Autodesk Inventor part; units mm, degrees
(part 6 of 6)
sketch "S15_195p3" plane through (0, 0, 0) normal (0, 0, 1) x (1, 0, 0)
  spline S0 degree 4 poles (125.9816, -53.0872) (125.9571, -53.0702) (125.8376, -52.9864) (125.6366, -52.8466) (125.2975, -52.6104) (124.9408, -52.3617) (124.502, -52.0575) (123.9855, -51.6987) (123.3893, -51.2867) (122.7156, -50.8212) (121.9638, -50.3042) (121.135, -49.7351) (120.2298, -49.1159) (119.2485, -48.447) (118.1926, -47.7295) (117.0618, -46.9649) (115.8579, -46.154) (114.5815, -45.2984) (113.2337, -44.3985) (111.8153, -43.4568) (110.3277, -42.474) (108.772, -41.4519) (107.1492, -40.3915) (105.4613, -39.2947) (103.7089, -38.1629) (101.8941, -36.9982) (100.0179, -35.8012) (98.0825, -34.5747) (96.0888, -33.3192) (94.0391, -32.0378) (91.9348, -30.7309) (89.7779, -29.4013) (87.5702, -28.05) (85.3138, -26.6795) (83.0104, -25.2909) (80.6627, -23.8865) (78.2717, -22.4682) (75.8404, -21.0375) (73.3708, -19.5968) (70.865, -18.1474) (68.3252, -16.6917) (65.7538, -15.2313) (63.1532, -13.7681) (60.5259, -12.3041) (57.8736, -10.8415) (55.1998, -9.382) (52.5061, -7.927) (49.7953, -6.4797) (47.0699, -5.0405) (44.3326, -3.6125) (41.5854, -2.1967) (38.8317, -0.7957) (36.073, 0.5886) (33.3129, 1.9555) (30.5532, 3.3018) (27.7948, 4.6278) (25.0442, 5.9287) (22.2894, 7.2111) (19.5352, 8.4618) (16.7929, 9.679) (14.0628, 10.861) (11.3496, 12.0056) (8.6564, 13.1126) (5.9856, 14.1789) (3.3403, 15.2059) (0.7234, 16.1899) (-1.8626, 17.1321) (-4.4145, 18.0303) (-6.9297, 18.8849) (-9.4054, 19.6941) (-11.839, 20.4583) (-14.2276, 21.1764) (-16.5684, 21.8487) (-18.8593, 22.4742) (-21.097, 23.0535) (-23.2793, 23.5858) (-25.4039, 24.072) (-27.468, 24.5112) (-29.4695, 24.9047) (-31.4059, 25.2518) (-33.2754, 25.5529) (-35.0752, 25.8094) (-36.8039, 26.0205) (-38.4591, 26.1872) (-40.0392, 26.3106) (-41.5422, 26.3902) (-42.9667, 26.4274) (-44.3109, 26.4227) (-45.5737, 26.3765) (-46.7533, 26.2893) (-47.8492, 26.1622) (-48.8598, 25.9957) (-49.7845, 25.7897) (-50.623, 25.546) (-51.3739, 25.263) (-52.0377, 24.9422) (-52.6135, 24.5832) (-53.1006, 24.185) (-53.497, 23.7471) (-53.8017, 23.2714) (-54.0117, 22.7577) (-54.1273, 22.2149) (-54.1441, 21.6505) (-54.0641, 21.0658) (-53.8887, 20.4629) (-53.6195, 19.8419) (-53.2579, 19.2032) (-52.805, 18.5459) (-52.2615, 17.8703) (-51.628, 17.1764) (-50.9052, 16.4646) (-50.094, 15.7355) (-49.1952, 14.9891) (-48.2099, 14.2264) (-47.1391, 13.4475) (-45.984, 12.6535) (-44.7459, 11.8441) (-43.4261, 11.0212) (-42.0259, 10.1841) (-40.5473, 9.334) (-38.9911, 8.4715) (-37.3595, 7.5976) (-35.6542, 6.7113) (-33.8766, 5.8153) (-32.0292, 4.9082) (-30.113, 3.9916) (-28.131, 3.0654) (-26.0847, 2.1299) (-23.9762, 1.1866) (-21.808, 0.2339) (-19.5818, -0.7255) (-17.3006, -1.6936) (-14.9662, -2.6682) (-12.581, -3.6503) (-10.1481, -4.6394) (-7.6689, -5.6346) (-5.1471, -6.6365) (-2.5846, -7.6445) (0.0159, -8.6582) (2.6516, -9.6779) (5.3196, -10.7034) (8.0177, -11.7337) (10.7442, -12.7705) (13.4952, -13.8109) (16.2737, -14.861) (19.0868, -15.914) (21.9144, -16.9645) (24.7602, -18.013) (27.6171, -19.0583) (30.4832, -20.1002) (33.3552, -21.1382) (36.2298, -22.1711) (39.1042, -23.1993) (41.9758, -24.221) (44.841, -25.2372) (47.6974, -26.2455) (50.5415, -27.247) (53.3708, -28.2398) (56.1826, -29.2234) (58.9732, -30.1979) (61.7404, -31.1616) (64.4815, -32.1139) (67.1932, -33.055) (69.873, -33.9827) (72.5183, -34.8976) (75.1261, -35.798) (77.6941, -36.6833) (80.2194, -37.5527) (82.6998, -38.4058) (85.1322, -39.2415) (87.5148, -40.0589) (89.845, -40.8572) (92.1199, -41.6363) (94.3379, -42.3942) (96.4964, -43.1316) (98.5933, -43.8466) (100.6262, -44.5396) (102.5936, -45.2086) (104.4929, -45.8543) (106.3223, -46.4752) (108.0801, -47.0711) (109.7642, -47.641) (111.373, -48.1854) (112.905, -48.7023) (114.3582, -49.1926) (115.7313, -49.6552) (117.023, -50.0894) (118.2315, -50.4956) (119.356, -50.8732) (120.395, -51.2212) (121.3472, -51.5403) (122.2122, -51.8294) (122.9882, -52.0891) (123.6752, -52.3183) (124.2717, -52.5174) (124.7779, -52.6863) (125.1907, -52.8235) (125.5826, -52.9546) (125.815, -53.0316) (125.9533, -53.0777) (125.9816, -53.0872) knots 0 0 0 0 0 0.003306 0.005253 0.00752 0.010062 0.01285 0.015861 0.019079 0.022488 0.026078 0.029837 0.033757 0.037828 0.042045 0.046398 0.050884 0.055494 0.060224 0.065069 0.070023 0.075082 0.080241 0.085495 0.090841 0.096274 0.101791 0.107386 0.113057 0.118799 0.124609 0.130484 0.136419 0.142412 0.148458 0.154554 0.160697 0.166884 0.17311 0.179374 0.185671 0.191998 0.198352 0.20473 0.211128 0.217543 0.223972 0.230412 0.23686 0.243312 0.249765 0.256217 0.262663 0.2691 0.275526 0.281941 0.288345 0.294734 0.301105 0.307451 0.313767 0.320049 0.326294 0.332498 0.338659 0.344773 0.350837 0.356848 0.362801 0.368695 0.374525 0.380288 0.38598 0.391599 0.39714 0.4026 0.407976 0.413263 0.418458 0.423557 0.428556 0.433452 0.438241 0.442917 0.447478 0.451919 0.456236 0.460425 0.464482 0.468403 0.472185 0.475825 0.479322 0.482675 0.485889 0.48897 0.49193 0.494788 0.497572 0.50031 0.503032 0.505769 0.508552 0.511409 0.514365 0.517441 0.520647 0.523991 0.527474 0.531098 0.534861 0.538758 0.542789 0.546947 0.551231 0.555634 0.560154 0.564786 0.569527 0.574371 0.579315 0.584356 0.58949 0.594712 0.60002 0.605409 0.610877 0.61642 0.622034 0.627716 0.633463 0.639271 0.645138 0.651061 0.657035 0.663059 0.669128 0.675241 0.681393 0.687582 0.693804 0.700057 0.706341 0.712655 0.718998 0.725365 0.731751 0.738149 0.744556 0.750969 0.757385 0.7638 0.770211 0.776616 0.783011 0.789393 0.795759 0.802106 0.808429 0.814727 0.820996 0.827232 0.833433 0.839595 0.845714 0.851788 0.857813 0.863785 0.869702 0.875558 0.881352 0.887078 0.892735 0.898316 0.90382 0.909242 0.914577 0.919822 0.924972 0.930023 0.93497 0.939808 0.944533 0.949139 0.95362 0.95797 0.962183 0.966252 0.970169 0.973927 0.977515 0.980924 0.984141 0.987151 0.989939 0.99248 0.994747 0.996694 1 1 1 1 1
  circle A0 centre (0, 0) radius 5.15
  line L0 (-27.08, 9.9) -> (-16.88, 9.9)
  line L1 (-16.88, 9.9) -> (-16.88, 14.1)
  line L2 (-16.88, 14.1) -> (-27.08, 14.1)
  line L3 (-27.08, 14.1) -> (-27.08, 9.9)
  line L4 (-27.08, 9.9) -> (-16.88, 14.1) construction
  line L5 (-16.88, 9.9) -> (-27.08, 14.1) construction
  line L6 (40.1, -9) -> (29.9, -9)
  line L7 (29.9, -9) -> (29.9, -13.2)
  line L8 (29.9, -13.2) -> (40.1, -13.2)
  line L9 (40.1, -13.2) -> (40.1, -9)
  line L10 (40.1, -9) -> (29.9, -13.2) construction
  line L11 (29.9, -9) -> (40.1, -13.2) construction
  point P0 (125.8216, -52.9755)
  point P1 (125.6216, -52.8361)
  point P2 (125.3419, -52.6413)
  point P3 (124.9828, -52.3912)
  point P4 (124.5442, -52.0867)
  point P5 (124.0266, -51.7276)
  point P6 (123.4303, -51.3151)
  point P7 (122.7559, -50.8495)
  point P8 (122.0038, -50.3318)
  point P9 (121.1745, -49.7626)
  point P10 (120.2687, -49.1429)
  point P11 (119.287, -48.4737)
  point P12 (118.2303, -47.7559)
  point P13 (117.0991, -46.9907)
  point P14 (115.8945, -46.1794)
  point P15 (114.6175, -45.3232)
  point P16 (113.269, -44.4231)
  point P17 (111.8498, -43.4807)
  point P18 (110.3614, -42.4974)
  point P19 (108.8049, -41.4747)
  point P20 (107.1814, -40.4137)
  point P21 (105.4925, -39.3163)
  point P22 (103.7393, -38.184)
  point P23 (101.9236, -37.0185)
  point P24 (100.0465, -35.8211)
  point P25 (98.1099, -34.5937)
  point P26 (96.1153, -33.3377)
  point P27 (94.0645, -32.0555)
  point P28 (91.9591, -30.748)
  point P29 (89.8011, -29.4175)
  point P30 (87.5924, -28.0657)
  point P31 (85.3348, -26.6943)
  point P32 (83.0303, -25.3051)
  point P33 (80.6812, -23.9)
  point P34 (78.2891, -22.4809)
  point P35 (75.8565, -21.0495)
  point P36 (73.3857, -19.608)
  point P37 (70.8786, -18.158)
  point P38 (68.3375, -16.7015)
  point P39 (65.7647, -15.2403)
  point P40 (63.1628, -13.7764)
  point P41 (60.534, -12.3118)
  point P42 (57.8805, -10.8484)
  point P43 (55.2052, -9.3881)
  point P44 (52.5101, -7.9326)
  point P45 (49.7979, -6.4844)
  point P46 (47.0711, -5.0447)
  point P47 (44.3323, -3.616)
  point P48 (41.5838, -2.1997)
  point P49 (38.8284, -0.798)
  point P50 (36.0685, 0.5871)
  point P51 (33.3069, 1.9542)
  point P52 (30.5459, 3.3012)
  point P53 (27.7884, 4.6264)
  point P54 (25.0368, 5.9279)
  point P55 (22.2802, 7.2088)
  point P56 (19.5233, 8.4612)
  point P57 (16.7777, 9.6794)
  point P58 (14.0462, 10.8618)
  point P59 (11.3315, 12.007)
  point P60 (8.6368, 13.1139)
  point P61 (5.9647, 14.181)
  point P62 (3.318, 15.2077)
  point P63 (0.6997, 16.1923)
  point P64 (-1.8875, 17.1344)
  point P65 (-4.4407, 18.0329)
  point P66 (-6.9572, 18.8874)
  point P67 (-9.4342, 19.6968)
  point P68 (-11.8691, 20.4608)
  point P69 (-14.2588, 21.179)
  point P70 (-16.6008, 21.8509)
  point P71 (-18.8928, 22.4764)
  point P72 (-21.1316, 23.0553)
  point P73 (-23.3149, 23.5875)
  point P74 (-25.4404, 24.073)
  point P75 (-27.5056, 24.512)
  point P76 (-29.5079, 24.9048)
  point P77 (-31.4452, 25.2513)
  point P78 (-33.3153, 25.5519)
  point P79 (-35.1159, 25.8073)
  point P80 (-36.8451, 26.0175)
  point P81 (-38.5008, 26.1833)
  point P82 (-40.0812, 26.3052)
  point P83 (-41.5845, 26.3837)
  point P84 (-43.0089, 26.4193)
  point P85 (-44.3529, 26.4128)
  point P86 (-45.6152, 26.3646)
  point P87 (-46.794, 26.2754)
  point P88 (-47.8885, 26.146)
  point P89 (-48.8972, 25.9768)
  point P90 (-49.8192, 25.7683)
  point P91 (-50.6537, 25.5214)
  point P92 (-51.3998, 25.2362)
  point P93 (-52.0569, 24.9136)
  point P94 (-52.6244, 24.554)
  point P95 (-53.1019, 24.1576)
  point P96 (-53.489, 23.7248)
  point P97 (-53.7859, 23.2561)
  point P98 (-53.9921, 22.7517)
  point P99 (-54.1059, 22.2187)
  point P100 (-54.125, 21.6643)
  point P101 (-54.05, 21.0889)
  point P102 (-53.8812, 20.4926)
  point P103 (-53.619, 19.8758)
  point P104 (-53.2638, 19.2391)
  point P105 (-52.8162, 18.5825)
  point P106 (-52.2772, 17.9068)
  point P107 (-51.6474, 17.2122)
  point P108 (-50.9275, 16.4994)
  point P109 (-50.1186, 15.769)
  point P110 (-49.2216, 15.0214)
  point P111 (-48.2377, 14.2573)
  point P112 (-47.1679, 13.4772)
  point P113 (-46.0136, 12.6818)
  point P114 (-44.776, 11.8714)
  point P115 (-43.4565, 11.0471)
  point P116 (-42.0566, 10.209)
  point P117 (-40.5778, 9.3578)
  point P118 (-39.0216, 8.4943)
  point P119 (-37.3897, 7.6191)
  point P120 (-35.684, 6.7323)
  point P121 (-33.9061, 5.835)
  point P122 (-32.0581, 4.9272)
  point P123 (-30.1415, 4.0095)
  point P124 (-28.1587, 3.0825)
  point P125 (-26.1117, 2.1464)
  point P126 (-24.0026, 1.2018)
  point P127 (-21.8334, 0.2488)
  point P128 (-19.6065, -0.7119)
  point P129 (-17.3243, -1.6803)
  point P130 (-14.989, -2.6559)
  point P131 (-12.6029, -3.6387)
  point P132 (-10.1688, -4.6284)
  point P133 (-7.6887, -5.6245)
  point P134 (-5.1658, -6.627)
  point P135 (-2.6021, -7.6357)
  point P136 (-0.0005, -8.6502)
  point P137 (2.6364, -9.6706)
  point P138 (5.3056, -10.6967)
  point P139 (8.0047, -11.7278)
  point P140 (10.7308, -12.7643)
  point P141 (13.4812, -13.8054)
  point P142 (16.2622, -14.8546)
  point P143 (19.0767, -15.9086)
  point P144 (21.9086, -16.9605)
  point P145 (24.7556, -18.0098)
  point P146 (27.6142, -19.0558)
  point P147 (30.4816, -20.0984)
  point P148 (33.355, -21.1369)
  point P149 (36.2311, -22.1706)
  point P150 (39.107, -23.1991)
  point P151 (41.9798, -24.2218)
  point P152 (44.8466, -25.2382)
  point P153 (47.7044, -26.2475)
  point P154 (50.55, -27.2493)
  point P155 (53.3807, -28.2427)
  point P156 (56.1939, -29.227)
  point P157 (58.986, -30.2018)
  point P158 (61.7546, -31.1661)
  point P159 (64.497, -32.1191)
  point P160 (67.2103, -33.0604)
  point P161 (69.8914, -33.9889)
  point P162 (72.538, -34.9041)
  point P163 (75.1473, -35.805)
  point P164 (77.7165, -36.6908)
  point P165 (80.2432, -37.5607)
  point P166 (82.7249, -38.4143)
  point P167 (85.1586, -39.2503)
  point P168 (87.5424, -40.0681)
  point P169 (89.8738, -40.867)
  point P170 (92.15, -41.6463)
  point P171 (94.3691, -42.4048)
  point P172 (96.5288, -43.1424)
  point P173 (98.6268, -43.8579)
  point P174 (100.6608, -44.5511)
  point P175 (102.6292, -45.2207)
  point P176 (104.5295, -45.8665)
  point P177 (106.3599, -46.4878)
  point P178 (108.1187, -47.084)
  point P179 (109.8037, -47.6544)
  point P180 (111.4134, -48.1987)
  point P181 (112.9462, -48.7162)
  point P182 (114.4002, -49.2066)
  point P183 (115.7741, -49.6694)
  point P184 (117.0664, -50.104)
  point P185 (118.2757, -50.5104)
  point P186 (119.4009, -50.8881)
  point P187 (120.4404, -51.2365)
  point P188 (121.3934, -51.5556)
  point P189 (122.2588, -51.845)
  point P190 (123.0355, -52.1047)
  point P191 (123.7229, -52.3342)
  point P192 (124.3203, -52.5336)
  point P193 (124.8266, -52.7024)
  point P194 (125.242, -52.8408)
  point P195 (125.5653, -52.9487)
  point P196 (125.7965, -53.0255)
  point P197 (125.9354, -53.0718)
  point P198 (-21.98, 12)
  point P199 (35, -11.1)
  dimension "d29" = 10.3
  dimension "d30" = 58.59
  dimension "d125" = 10.2
  dimension "d126" = 4.2
  dimension "d182" = 21.98
  dimension "d183" = 12
  dimension "d299" = 10.2
  dimension "d300" = 4.2
  dimension "d301" = 35
  dimension "d302" = 11.1
  constraints: 24 end point, 4 midpoint, 4 parallel, 2 horizontal, 2 perpendicular, 1 centre point, 201 other
  measures "d29" diameter of A0
  measures "d30" distance of A0.centre point (-53.992, 22.752)
  measures "d125" distance of L2.end L1.end
  measures "d126" distance of L1.end L0.end
  measures "d182" horizontal distance of point (0, 0) point (-21.98, 12)
  measures "d183" vertical distance of point (0, 0) point (-21.98, 12)
  measures "d299" distance of L8.end L7.end
  measures "d300" distance of L7.end L6.end
  measures "d301" horizontal distance of point (35, -11.1) point (0, 0)
  measures "d302" vertical distance of point (0, 0) point (35, -11.1)
extrude "Extrusion1" add sketch "S01_282p7" along normal blind 3
extrude "Extrusion2" add sketch "S02_317p9" against normal blind 3 separate body
extrude "Extrusion3" add sketch "S03_340p2" along normal blind 3 separate body
move or copy body "Move Body3" bodies to move or copy 3 copy no translate (0, 0, -30)
extrude "Extrusion4" add sketch "S04_341p5" along normal blind 3 separate body
move or copy body "Move Body4" bodies to move or copy 4 copy no translate (0, 0, -45)
extrude "Extrusion5" add sketch "S05_329p0" along normal blind 3 separate body
move or copy body "Move Body5" bodies to move or copy 5 copy no translate (0, 0, -60)
extrude "Extrusion6" add sketch "S06_305p5" along normal blind 3 separate body
move or copy body "Move Body6" bodies to move or copy 6 copy no translate (0, 0, -75)
extrude "Extrusion7" add sketch "S07_285p6" along normal blind 3 separate body
move or copy body "Move Body7" bodies to move or copy 7 copy no translate (0, 0, -90)
extrude "Extrusion8" add sketch "S08_271p4" along normal blind 3 separate body
move or copy body "Move Body8" bodies to move or copy 8 copy no translate (0, 0, -105)
extrude "Extrusion9" add sketch "S09_267p4" along normal blind 3 separate body
move or copy body "Move Body9" bodies to move or copy 9 copy no translate (0, 0, -120)
extrude "Extrusion10" add sketch "S10_259p0" along normal blind 3 separate body
move or copy body "Move Body10" bodies to move or copy 10 copy no translate (0, 0, -135)
extrude "Extrusion11" add sketch "S11_257p6" along normal blind 3 separate body
move or copy body "Move Body11" bodies to move or copy 11 copy no translate (0, 0, -150)
extrude "Extrusion12" add sketch "S12_252p5" along normal blind 3 separate body
move or copy body "Move Body12" bodies to move or copy 12 copy no translate (0, 0, -165)
extrude "Extrusion13" add sketch "S13_240p0" along normal blind 3 separate body
move or copy body "Move Body13" bodies to move or copy 13 copy no translate (0, 0, -180)
extrude "Extrusion14" add sketch "S14_219p8" along normal blind 3 separate body
move or copy body "Move Body14" bodies to move or copy 14 copy no translate (0, 0, -195)
extrude "Extrusion15" add sketch "S15_195p3" along normal blind 3 separate body
move or copy body "Move Body15" bodies to move or copy 15 copy no translate (0, 0, -210)
move or copy body "Move Body16" bodies to move or copy 2 copy no translate (0, 0, -18)
move or copy body "Move Body17" bodies to move or copy 2 copy no translate (0, 0, 5)
body "Solid1"
body "Solid2"
body "Solid3"
body "Solid4"
body "Solid5"
body "Solid6"
body "Solid7"
body "Solid8"
body "Solid9"
body "Solid10"
body "Solid11"
body "Solid12"
body "Solid13"
body "Solid14"
body "Solid15"
